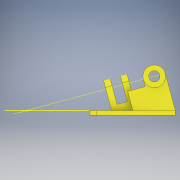
# Autodesk Inventor part: Reper
Saved by Autodesk Inventor 2019 (Build 230136000, 136)
## iProperties
Created: 2019-02-26
Part Number: Reper
Material: Steel, Carbon
Document SubType Name: Modeling
Designer: forev
Density: 7.85 g/cm^3
Appearance: Canary
Mass: 882.58 g
Surface Area: 389.341 cm^2
Volume: 112.431 cm^3
Author: forev
Autodesk Inventor part; units mm, degrees
ref_plane "YZ Plane" through (0, 0, 0) normal (1, 0, 0) x (0, 1, 0)
ref_plane "XZ Plane" through (0, 0, 0) normal (0, 1, 0) x (-1, 0, 0)
ref_plane "XY Plane" through (0, 0, 0) normal (0, 0, 1) x (1, 0, 0)
sketch "Sketch1" plane through (0, 0, 0) normal (0, 0, 1) x (1, 0, 0)
  line L0 (-28.9877, 0) -> (173.9264, 0) projected
  line L1 (-29.4372, -7.8877) -> (176.6233, 47.3261) projected
  line L2 (101.2142, 39.5436) -> (111.8098, 0)
  line L3 (111.8098, 0) -> (144.9387, 0)
  line L4 (144.9387, 0) -> (132.1238, 47.8258)
  line L5 (132.1238, 47.8258) -> (123.4305, 45.4964)
  line L6 (123.4305, 45.4964) -> (132.4891, 11.689)
  line L7 (109.9075, 41.8729) -> (118.9662, 8.0655)
  line L8 (118.9662, 8.0655) -> (132.4891, 11.689)
  line L9 (109.9075, 41.8729) -> (101.2142, 39.5436)
  point P0 (0, 0)
  point P1 (132.0574, 26.729)
  point P2 (96.5926, 25.8819)
  dimension "d0" = 12
  dimension "d1" = 9
  dimension "d2" = 14
  dimension "d3" = 9
  dimension "d4" = 35
  dimension "d5" = 117
  constraints: 16 end point, 3 perpendicular, 2 collinear, 2 parallel, 1 horizontal
  measures "d0" distance between parallel lines of L1 L5
  measures "d1" distance between parallel lines of L2 L7
  measures "d2" distance between parallel lines of L6 L7
  measures "d3" distance between parallel lines of L4 L6
  measures "d4" distance between parallel lines of L8 L9
  measures "d5" distance from line of point (0, 0) L7
extrude "Extrusion1" add sketch "Sketch1" along normal mid plane 50 contours L2 L1 L7 L8 L6 L4 L0 | L2 L9 L7 L1 | L1 L6 L5 L4
sketch "Sketch3" plane through (111.8098, 0, -25) normal (-0.9659, -0.2588, 0) x (0, 0, 1)
  line L0 (25, 64.8401) -> (25, -46.4712) projected
  line L1 (50, 40.9385) -> (0, 40.9385) projected
  line L2 (50, -8.5744) -> (0, -8.5744) projected
  line L3 (50, 40.9385) -> (0, 40.9385) projected
  line L4 (1.57, -23.5744) -> (48.43, -23.5744)
  line L5 (1.57, -23.5744) -> (13.2622, 31.4335)
  line L6 (48.43, -23.5744) -> (36.7378, 31.4335)
  arc A0 (36.7378, 31.4335) -> (13.2622, 31.4335) centre (25, 28.9385) ccw
  dimension "d8" = 12
  dimension "d9" = 78
  dimension "d10" = 78
  dimension "d12" = 15
  constraints: 6 end point, 3 tangent, 2 point on circle, 1 centre point, 1 horizontal, 1 point on line
  measures "d8" radius of A0
  measures "d9" angle of L4 L5
  measures "d10" angle of L4 L6
  measures "d12" distance between parallel lines of L4 L2
extrude "Extrusion2" cut sketch "Sketch3" against normal through all keep common part
sketch "Sketch4" plane through (0, 0, 0) normal (0, 0, 1) x (1, 0, 0)
  point P0 (0, 0)
sketch "Sketch5" plane through (0, 0, 0) normal (0, 0, 1) x (1, 0, 0)
  point P0 (0, 0)
sketch "Sketch6" plane through (0, 0, 0) normal (0, 0, 1) x (1, 0, 0)
  line L0 (-28.9877, 0) -> (173.9264, 0) projected
  point P0 (0, 0)
sketch "Sketch7" plane through (0, 0, 0) normal (0, 0, 1) x (1, 0, 0)
  line L0 (-28.9877, 0) -> (173.9264, 0) projected
  line L1 (-29.4372, -7.8877) -> (176.6233, 47.3261) projected
  line L2 (132.9832, 25.3) -> (139.7623, 0)
  line L3 (139.7623, 0) -> (195.6672, 0)
  line L4 (195.6672, 0) -> (182.56, 48.9168)
  line L5 (182.56, 48.9168) -> (153.5822, 41.1522)
  line L6 (153.5822, 41.1522) -> (156.1654, 31.5117)
  line L7 (156.1654, 31.5117) -> (132.9832, 25.3)
  line L8 (134.5839, 38.6446) -> (144.9387, 0) projected
  line L9 (132.1238, 47.8258) -> (134.5839, 38.6446) projected
  point P0 (0, 0)
  dimension "d15" = 5
  dimension "d16" = 49
  dimension "d17" = 30
  dimension "d18" = 25.3
  constraints: 12 end point, 4 perpendicular, 2 collinear, 1 horizontal
  measures "d15" distance between parallel lines of L2 L8
  measures "d16" distance between parallel lines of L4 L9
  measures "d17" distance between parallel lines of L4 L6
  measures "d18" distance from line of L2.start L0
extrude "Extrusion3" add sketch "Sketch7" along normal mid plane 61 contours L2 L7 L8 L0 | L8 L7 L6 L1 L5 L4 L3 L0
sketch "Sketch8" plane through (153.5822, 41.1522, 30.5) normal (-0.2588, 0.9659, 0) x (0.9659, 0.2588, 0)
  line L0 (-19, 56) -> (35, 56)
  line L1 (35, 56) -> (35, 5)
  line L2 (35, 5) -> (-19, 5)
  line L3 (-19, 5) -> (-19, 56)
  line L4 (0, 61) -> (30, 61) projected
  line L5 (30, 61) -> (30, 0) projected
  line L6 (30, 0) -> (0, 0) projected
  line L7 (0, 61) -> (0, 0) projected
  line L8 (-24, 0) -> (-24, 16.1105) projected
  line L9 (-24, 61) -> (0, 61) projected
  point P0 (-159, 30.5)
  dimension "d23" = 5
  dimension "d25" = 5
  dimension "d26" = 5
  dimension "d28" = 5
  constraints: 8 end point, 2 parallel, 1 horizontal, 1 perpendicular
  measures "d23" distance between parallel lines of L6 L2
  measures "d25" distance between parallel lines of L8 L3
  measures "d26" distance between parallel lines of L0 L9
  measures "d28" distance between parallel lines of L5 L1
extrude "Extrusion4" cut sketch "Sketch8" against normal through all contours L0 L7 L2 L3 | L0 L5 L2 L7 | L0 L1 L2 L5
sketch "Sketch9" plane through (0, 0, 0) normal (0, 0, 1) x (1, 0, 0)
  line L0 (153.5822, 41.1522) -> (182.56, 48.9168) projected
  line L1 (182.56, 48.9168) -> (195.6672, 0) projected
  line L2 (-39.5137, -10.5877) -> (237.0823, 63.526) projected
  line L3 (195.6672, 0) -> (182.56, 48.9168) projected
  line L4 (182.56, 48.9168) -> (153.5822, 41.1522) projected
  circle A0 centre (168.0711, 45.0345) radius 15
  point P0 (0, 0)
  dimension "d81" = 30
  constraints: 6 midpoint, 1 centre point, 1 coincident
  measures "d81" diameter of A0
extrude "Extrusion5" add sketch "Sketch9" along normal mid plane 71
sketch "Sketch11" plane through (0, 0, 0) normal (0, 0, 1) x (1, 0, 0)
  circle A0 centre (168.0711, 45.0345) radius 19.5
  circle A1 centre (168.0711, 45.0345) radius 15 projected
  point P0 (0, 0)
  dimension "d36" = 39
  constraints: 1 centre point, 1 concentric
  measures "d36" diameter of A0
extrude "Extrusion6" cut sketch "Sketch11" along normal mid plane 41 contours A0 | A1
sketch "Sketch12" plane through (0, 0, 0) normal (0, 1, 0) x (-1, 0, 0)
  line L0 (-234.8006, 0) -> (39.1334, 0) projected
  line L1 (-195.6672, -30.5) -> (-195.6672, 30.5)
  line L2 (-195.6672, 30.5) -> (-91.6172, 42.9434)
  line L3 (-82.6672, 35) -> (-82.6672, -35)
  line L4 (-91.6172, -42.9434) -> (-195.6672, -30.5)
  arc A0 (-91.6172, -42.9434) -> (-82.6672, -35) centre (-90.6672, -35) ccw
  arc A1 (-82.6672, 35) -> (-91.6172, 42.9434) centre (-90.6672, 35) ccw
  point P0 (0, 0)
  dimension "d39" = 8
  dimension "d40" = 8
  dimension "d41" = 113
  dimension "d42" = 70
  dimension "d43" = 35
  constraints: 8 end point, 4 point on circle, 4 tangent, 2 centre point, 1 coincident, 1 parallel, 1 vertical
  measures "d39" radius of A0
  measures "d40" radius of A1
  measures "d41" distance between parallel lines of L1 L3
  measures "d42" distance of L3.start L3.end
  measures "d43" distance from line of L0 L3.end
extrude "Extrusion7" add sketch "Sketch12" against normal blind 6
sketch "Sketch14" plane through (168.0711, 45.0345, -20.5) normal (0, 0, 1) x (1, 0, 0)
  circle A0 centre (0, 0) radius 15 projected
  point P0 (-168.0711, -45.0345)
  constraints: 1 coincident
hole "Hole1" at (168.0711, 45.0345, -20.5) direction (0, 0, -1) diameter 15 end through all
sketch "Sketch15" plane through (168.0711, 45.0345, 35.5) normal (0, 0, 1) x (1, 0, 0)
  circle A0 centre (0, 0) radius 15 projected
  point P0 (-168.0711, -45.0345)
  constraints: 1 coincident
hole "Hole2" at (168.0711, 45.0345, 35.5) direction (0, 0, -1) diameter 15 end through all
sketch "Sketch16" plane through (0, 0, 0) normal (0, 1, 0) x (1, 0, 0)
  arc A0 (91.6172, 42.9434) -> (82.6672, 35) centre (90.6672, 35) ccw projected
  point P0 (0, 0)
  constraints: 1 coincident
hole "Hole3" at (90.6672, 0, -35) direction (0, -1, 0) diameter 8 end through all
sketch "Sketch17" plane through (0, 0, 0) normal (0, 1, 0) x (1, 0, 0)
  arc A0 (82.6672, -35) -> (91.6172, -42.9434) centre (90.6672, -35) ccw projected
  point P0 (0, 0)
  constraints: 1 coincident
hole "Hole4" at (90.6672, 0, 35) direction (0, -1, 0) diameter 8 end through all
sketch "Sketch18" plane through (104.32, 27.9525, 0) normal (-0.9659, -0.2588, 0) x (0, 0, 1)
  arc A0 (11.7378, 2.4949) -> (-11.7378, 2.4949) centre (0, 0) ccw projected
  point P0 (0, 0)
  constraints: 1 coincident
hole "Hole5" at (104.32, 27.9525, 0) direction (0.9659, 0.2588, 0) diameter 9 end through all
equation "\"d81\" = d17"
equation "\"d36\" = 1.3 * d17"
equation "\"d43\" = 0.5 * d42"
body "Solid1"
